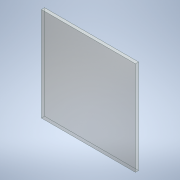
# Autodesk Inventor part: 00_Mirror_30x30
Saved by Autodesk Inventor 2022.3 (Build 263350000, 350)
## iProperties
Created: 2020-05-12
Part Number: 00_Mirror_30x30
Material: Glass
Document SubType Name: Modeling
Designer: B
Density: 2.18 g/cm^3
Appearance: Clear
Author: B
Autodesk Inventor part; units mm, degrees
ref_plane "YZ Plane" through (0, 0, 0) normal (1, 0, 0) x (0, 1, 0)
ref_plane "XZ Plane" through (0, 0, 0) normal (0, 1, 0) x (-1, 0, 0)
ref_plane "XY Plane" through (0, 0, 0) normal (0, 0, 1) x (1, 0, 0)
sketch "Sketch1" plane through (0, 0, 0) normal (0, 0, 1) x (1, 0, 0)
  line L0 (31, -30) -> (0, -30) construction
  line L1 (31, 0) -> (31, -30) construction
  line L2 (0, 0) -> (31, 0) construction
  line L3 (0, 0) -> (0, -30) construction
  line L4 (0.5676, 0) -> (30.5676, 0)
  line L5 (30.5676, 0) -> (30.5676, -30)
  line L6 (30.5676, -30) -> (0.5676, -30)
  line L7 (0.5676, -30) -> (0.5676, 0)
  dimension "d0" = 30
  constraints: 8 end point, 2 parallel, 2 point on line, 1 horizontal, 1 perpendicular
  measures "d0" distance between parallel lines of L5 L7
extrude "Extrusion1" add sketch "Sketch1" along normal blind 1
body "Solid1"
